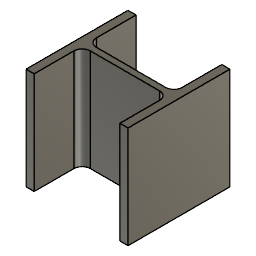
H-100×100×6×8 (Autodesk Fusion 360 design; units mm, degrees)
Autodesk Fusion 360 part; units mm, degrees
sketch "スケッチ1" plane through (0, 0, 0) normal (0, 0, 1) x (1, 0, 0)
  line L0 (0, 50) -> (0, -50)
  line L1 (100, -50) -> (100, 50)
  line L2 (8, -50) -> (8, -11)
  line L3 (0, -50) -> (8, -50)
  line L4 (92, -11) -> (92, -50)
  line L5 (92, -50) -> (100, -50)
  line L6 (84, 3) -> (16, 3)
  line L7 (16, -3) -> (84, -3)
  line L8 (8, 11) -> (8, 50)
  line L9 (8, 50) -> (0, 50)
  line L10 (92, 50) -> (92, 11)
  line L11 (100, 50) -> (92, 50)
  arc A0 (16, -3) -> (8, -11) centre (16, -11) ccw
  arc A1 (8, 11) -> (16, 3) centre (16, 11) ccw
  arc A2 (84, 3) -> (92, 11) centre (84, 11) ccw
  arc A3 (92, -11) -> (84, -3) centre (84, -11) ccw
extrude "押し出し1" add sketch "スケッチ1" along normal blind 100
